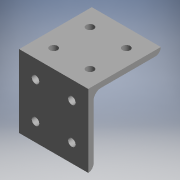
# Autodesk Inventor part: 40-4304 Aluminum
Saved by Autodesk Inventor 2017.3 (Build 213256000, 256)
## iProperties
Part Number: 40-4304 Aluminum
Material: Generic
Catalog Web Link: www.cadenas.de
Description: 25-4114, 40-4304, 45-4304, 25-4114-Black, 40-4304-Black, 45-4304-Black-8 Hole Inside Corner Bracket
Vendor: 8020
Document SubType Name: Modeling
Designer: partserver
Manufacturer: 8020
Mass: 67.4964 g
Surface Area: 258.981 cm^2
Volume: 67.4964 cm^3
Density: 1 g/cm^3
Appearance: PSOLRGB-191-191-191
Category: PARTsolutions
Company: 8020
Title: 40-4304
Author: Cadenas PARTsolutions
Comments: 8 Hole Inside Corner Bracket
PSOL_IDENT_0: {$CADENAS_DATA\23d-libs\8020\metric\joining_plates\25_4114.prj},218 {VTYP=3D},{NB=40-4304},{LINA=40-
PSOL_IDENT_1: 4304},{NN=25-4114, 40-4304, 45-4304, 25-4114-Black, 40-4304-Black, 45-4304-Black},{DATE=31.07.2020 0
PSOL_IDENT_2: 9:21:28},{GEOMDATE=11.07.2018 13:40:00},{VERSION=},{LINEID=20},{WBVAR=},{WBNUMERIC=}  {NB=40-4304},{
PSOL_IDENT_3: LINA=40-4304},{KT=DUMMY},{PN=40-4304},{SERIES=40},{MATERIAL=Aluminum},{GRADE=6105-T5},{FINISH=Clear
PSOL_IDENT_4: Anodize},{A=76.00},{B=80.00},{C=80.00},{D=40.00},{E=8.30},{F=20.00},{G=18.00},{T=6.00},{W=.166},{C3=
PSOL_IDENT_5: 60.000},{R=8.000},{COLOR=.75,.75,.75}
NB: 40-4304
NN: 25-4114, 40-4304, 45-4304, 25-4114-Black, 40-4304-Black, 45-4304-Black
NT: 8 Hole Inside Corner Bracket
NBSYN: $PN.
LINA: 40-4304
CATALOG: 80/20
PN: 40-4304
SERIES: 40
MATERIAL: Aluminum
GRADE: 6105-T5
FINISH: Clear Anodize
A: 76
B: 80
C: 80
D: 40
E: 8.3
F: 20
G: 18
T: 6
W: .166
COLOR: .75,.75,.75
SUPPLIER: 8020
ARTICLENO: 40-4304
BOMINFO: 40-4304
CREATOR: CADENAS GmbH
Autodesk Inventor part; units mm, degrees
ref_plane "YZ Plane" through (0, 0, 0) normal (1, 0, 0) x (0, 1, 0)
ref_plane "XZ Plane" through (0, 0, 0) normal (0, 1, 0) x (-1, 0, 0)
ref_plane "XY Plane" through (0, 0, 0) normal (0, 0, 1) x (1, 0, 0)
sketch "Sketch_1" plane through (0, 0, 0) normal (1, 0, 0) x (0, 1, 0)
  line L0 (0, 80) -> (0, 0)
  line L1 (0, 0) -> (80, 0)
  arc A0 (80, 0) -> (74, 6) centre (74, 0) ccw
  line L2 (74, 6) -> (14, 6)
  arc A1 (6, 14) -> (14, 6) centre (14, 14) ccw
  line L3 (6, 14) -> (6, 74)
  arc A2 (6, 74) -> (0, 80) centre (0, 74) ccw
  constraints: 8 end point, 6 point on circle, 3 centre point
extrude "Extrusion1" add sketch "Sketch_1" along normal mid plane 76
sketch "Sketch2" plane through (38, 80, 0) normal (0, 0, -1) x (-1, 0, 0)
  point P0 (18, -20)
hole "Hole1" at (20, 60, 0) direction (0, 0, 1) diameter 8.3 depth 6.6
sketch "Sketch3" plane through (38, 80, 0) normal (0, 0, -1) x (-1, 0, 0)
  point P0 (58, -60)
hole "Hole2" at (-20, 20, 0) direction (0, 0, 1) diameter 8.3 depth 6.6
sketch "Sketch4" plane through (38, 80, 0) normal (0, 0, -1) x (-1, 0, 0)
  point P0 (58, -20)
hole "Hole3" at (-20, 60, 0) direction (0, 0, 1) diameter 8.3 depth 6.6
sketch "Sketch5" plane through (-38, 0, 0) normal (0, -1, 0) x (1, 0, 0)
  point P0 (58, 20)
hole "Hole4" at (20, 0, 20) direction (0, 1, 0) diameter 8.3 depth 6.6
sketch "Sketch6" plane through (-38, 0, 0) normal (0, -1, 0) x (1, 0, 0)
  point P0 (58, 60)
hole "Hole5" at (20, 0, 60) direction (0, 1, 0) diameter 8.3 depth 6.6
sketch "Sketch7" plane through (-38, 0, 0) normal (0, -1, 0) x (1, 0, 0)
  point P0 (18, 20)
hole "Hole6" at (-20, 0, 20) direction (0, 1, 0) diameter 8.3 depth 6.6
sketch "Sketch8" plane through (-38, 0, 0) normal (0, -1, 0) x (1, 0, 0)
  point P0 (18, 60)
hole "Hole7" at (-20, 0, 60) direction (0, 1, 0) diameter 8.3 depth 6.6
sketch "Sketch9" plane through (38, 80, 0) normal (0, 0, -1) x (-1, 0, 0)
  point P0 (18, -60)
hole "Hole8" at (20, 20, 0) direction (0, 0, 1) diameter 8.3 depth 6.6
body "Solid1"
